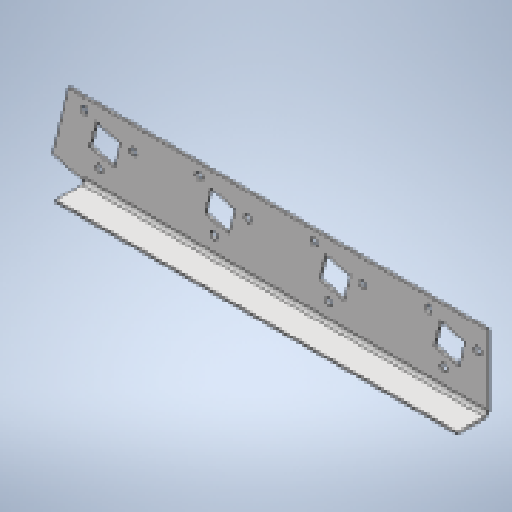
# Autodesk Inventor part: DSB-102 ridge bottom
Saved by Autodesk Inventor 2025.1 (Build 291241020, 241B)
## iProperties
Created: 2025-01-13
Part Number: DSB-102 ridge bottom
Material: Stainless Steel
Document SubType Name: Sheet Metal
Designer: user
Mass: 1273.74 g
Surface Area: 1640.62 cm^2
Volume: 159.218 cm^3
Density: 8 g/cm^3
Sheet Metal Rule: AISI304 3mm Die 32
Sheet Metal Width: 143.927 mm
Sheet Metal Length: 606.604 mm
Sheet Metal Area: 87306.942 mm^2
Appearance: Default
Flat Pattern Width: 14.3927 cm
Flat Pattern Length: 60.6604 cm
Flat Pattern Area: 873.069 cm^2
Author: user
Autodesk Inventor part; units mm, degrees
ref_plane "YZ Plane" through (0, 0, 0) normal (1, 0, 0) x (0, 1, 0)
ref_plane "XZ Plane" through (0, 0, 0) normal (0, 1, 0) x (-1, 0, 0)
ref_plane "XY Plane" through (0, 0, 0) normal (0, 0, 1) x (1, 0, 0)
sketch "Sketch1" plane through (0, 0, 0) normal (0, 0, 1) x (1, 0, 0)
  line L0 (0, -22.5) -> (560, -22.5)
  line L1 (560, -22.5) -> (560, 22.5)
  line L2 (560, 22.5) -> (0, 22.5)
  line L3 (0, 22.5) -> (0, -22.5)
  line L4 (0, -22.5) -> (560, 22.5) construction
  line L5 (560, -22.5) -> (0, 22.5) construction
  point P0 (0, 0)
  point P1 (0, 0)
  dimension "d154" = 560
  dimension "d155" = 45
  measures "d154" distance of L1.end L2.end
  measures "d155" distance of L0.end L1.end
extrude "Plate3" add sketch "Sketch1" along normal blind 3
sketch "Sketch7" plane through (0, 19.5, 0) normal (0, 1, 0) x (-1, 0, 0)
  line L0 (-560, 0) -> (0, 0)
  line L1 (0, 0) -> (0, 105)
  line L2 (0, 105) -> (-560, 105)
  line L3 (-560, 105) -> (-560, 0)
  constraints: 6 end point, 1 horizontal, 1 perpendicular, 1 vertical
edge flange "Flange3" height 105 angle 90 thickness 3 bend radius 5 thickness toward (0, 1, 0) relief round relief width 3 relief depth 1.5 edges at (280, 22.5, 3) wall of the first edge with corners at (560, 19.5, 0) (0, 19.5, 0) (0, 19.5, 105) (560, 19.5, 105)
bend "Bend3"
corner "Corner3"
sketch "Sketch11" plane through (0, 19.5, 105) normal (0, -1, 0) x (1, 0, 0)
  line L0 (0, -97) -> (560, -97) projected
  line L1 (560, -97) -> (560, 0) projected
  line L2 (560, 0) -> (0, 0) projected
  line L3 (0, -97) -> (0, 0) projected
  line L4 (0, 0) -> (-24.0074, 0)
  line L5 (-24.0074, 0) -> (-49.4388, -102)
  line L6 (-49.4388, -102) -> (-1, -102)
  line L7 (-1, -102) -> (-1, -97)
  line L8 (-1, -97) -> (0, -97)
  line L9 (560, -102) -> (0, -102) projected
  line L10 (-1, -102) -> (-46.6039, -90.6297)
  point P0 (0, -105)
  dimension "d193" = 1
  dimension "d194" = 24.0074
  dimension "d195" = 14
  dimension "d203" = 47
  constraints: 12 end point, 3 perpendicular, 1 collinear, 1 horizontal, 1 parallel, 1 point on line
  measures "d193" distance of L7.end L0.start
  measures "d194" distance of L2.end L4.end
  measures "d195" angle of L3 L5
  measures "d203" distance of L6.end L10.end
extrude "Extrusion6" add sketch "Sketch11" against normal up to surface (3 mm away) contours L8 L7 L10 L5 L4 L3
sketch "Sketch12" plane through (560, 19.5, 8) normal (0, -1, 0) x (1, 0, 0)
  line L0 (-511.7125, 66.6075) -> (-545.6729, 75.0748)
  line L1 (-545.6729, 75.0748) -> (-554.1401, 41.1144)
  line L2 (-554.1401, 41.1144) -> (-520.1798, 32.6472)
  line L3 (-520.1798, 32.6472) -> (-511.7125, 66.6075)
  line L4 (-511.7125, 66.6075) -> (-554.1401, 41.1144) construction
  line L5 (-545.6729, 75.0748) -> (-520.1798, 32.6472) construction
  circle A0 centre (-541.1517, 20.8709) radius 5.05
  circle A1 centre (-494.1275, 64.7996) radius 5.05
  circle A2 centre (-562.0482, 81.7341) radius 5.05
  line L6 (-494.1275, 64.7996) -> (-562.0482, 81.7341) construction
  line L7 (-562.0482, 81.7341) -> (-541.1517, 20.8709) construction
  line L8 (-541.1517, 20.8709) -> (-494.1275, 64.7996) construction
  line L9 (-528.6927, 70.8411) -> (-541.1517, 20.8709) construction
  line L10 (-584.0074, 97) -> (-606.6039, 6.3703) projected
  point P0 (-560, -8)
  point P1 (-532.9263, 53.861)
  point P2 (-544.0023, 9.4376)
  dimension "d206" = 35
  dimension "d207" = 35
  dimension "d208" = 10.1
  dimension "d209" = 70
  dimension "d210" = 54
  dimension "d211" = 20
  dimension "d213" = 12
  dimension "d214" = 60
  constraints: 20 end point, 4 parallel, 3 centre point, 3 midpoint, 1 equal radius, 1 perpendicular, 1 point on line, 2 other
  measures "d206" distance of L5.end L4.end
  measures "d207" distance of L4.end L5.start
  measures "d208" diameter of A0
  measures "d209" distance of L6.start L7.start
  measures "d210" distance from line of L9.end L6
  measures "d211" distance from line of L6 point (-532.926, 53.861)
  measures "d213" distance from line of L10.start L0
  measures "d214" distance from line of L10 point (-532.926, 53.861)
extrude "Cut1" cut sketch "Sketch12" against normal blind 3
pattern_linear "Rectangular Pattern5" count 4 spacing 160 along (1, 0, 0) of "Cut1"
body "Solid2"
